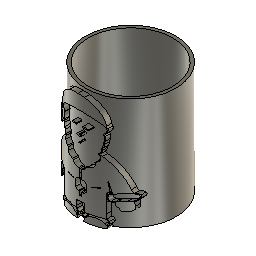
BICCHIERE BABBO NATALE v4 (Autodesk Fusion 360 design; units mm, degrees)
Autodesk Fusion 360 part; units mm, degrees
note: some values were not read from the file. Set by a fixed rule: which face or edge a step refers to.
(part 1 of 2)
sketch "Schizzo1" plane through (0, 0, 0) normal (0, 1, 0) x (1, 0, 0)
  spline S0 degree 3 poles (3.8329, -102.7667) (12.4583, -100.5971) (18.8877, -93.5063) (20.1048, -84.775) knots 0 0 0 0 1 1 1 1
  spline S1 degree 3 poles (20.1048, -84.775) (20.2635, -83.6902) (20.5281, -82.7377) (20.6869, -82.6319) knots 0 0 0 0 1 1 1 1
  spline S2 degree 3 poles (20.6869, -82.6319) (21.56, -82.1027) (21.0308, -79.7744) (19.7079, -78.2398) knots 0 0 0 0 1 1 1 1
  line L0 (19.7079, -78.2398) -> (18.7819, -77.155)
  line L1 (18.7819, -77.155) -> (19.1787, -75.885)
  spline S3 degree 3 poles (19.1787, -75.885) (19.6814, -74.2446) (19.6814, -73.4508) (19.2052, -72.0221) knots 0 0 0 0 1 1 1 1
  spline S4 degree 3 poles (19.2052, -72.0221) (18.9935, -71.3871) (18.7819, -70.17) (18.7554, -69.2969) knots 0 0 0 0 1 1 1 1
  spline S5 degree 3 poles (18.7554, -69.2969) (18.7289, -68.2121) (18.4908, -67.286) (18.041, -66.3865) knots 0 0 0 0 1 1 1 1
  spline S6 degree 3 poles (18.041, -66.3865) (17.6442, -65.6456) (17.406, -64.6931) (17.4325, -64.1904) knots 0 0 0 0 1 1 1 1
  spline S7 degree 3 poles (17.4325, -64.1904) (17.4854, -63.1321) (16.6387, -61.1213) (15.9244, -60.6715) knots 0 0 0 0 1 1 1 1
  spline S8 degree 3 poles (15.9244, -60.6715) (15.4217, -60.354) (15.5539, -60.2481) (17.3796, -59.1633) knots 0 0 0 0 1 1 1 1
  spline S9 degree 3 poles (17.3796, -59.1633) (24.3117, -55.1152) (29.9737, -45.9871) (33.1752, -33.7104) knots 0 0 0 0 1 1 1 1
  spline S10 degree 3 poles (33.1752, -33.7104) (33.8896, -31.0381) (34.1277, -30.4296) (34.4981, -30.4825) knots 0 0 0 0 1 1 1 1
  spline S11 degree 3 poles (34.4981, -30.4825) (35.1596, -30.6148) (36.3767, -29.6094) (36.9058, -28.551) knots 0 0 0 0 1 1 1 1
  spline S12 degree 3 poles (36.9058, -28.551) (37.4879, -27.2546) (37.2233, -25.72) (36.2179, -24.6881) knots 0 0 0 0 1 1 1 1
  spline S13 degree 3 poles (36.2179, -24.6881) (35.53, -23.9738) (35.1331, -23.7885) (34.551, -23.8944) knots 0 0 0 0 1 1 1 1
  spline S14 degree 3 poles (34.551, -23.8944) (34.4187, -23.9208) (34.3923, -23.4975) (34.4717, -22.9419) knots 0 0 0 0 1 1 1 1
  spline S15 degree 3 poles (34.4717, -22.9419) (34.5775, -22.3863) (34.7098, -20.9575) (34.8156, -19.7669) knots 0 0 0 0 1 1 1 1
  spline S16 degree 3 poles (34.8156, -19.7669) (35.0802, -16.5125) (34.6304, -16.0627) (30.6087, -15.5865) knots 0 0 0 0 1 1 1 1
  spline S17 degree 3 poles (30.6087, -15.5865) (29.18, -15.4277) (29.0477, -15.4542) (28.3333, -16.1685) knots 0 0 0 0 1 1 1 1
  spline S18 degree 3 poles (28.3333, -16.1685) (27.8571, -16.6448) (27.5131, -17.3592) (27.3808, -18.0471) knots 0 0 0 0 1 1 1 1
  spline S19 degree 3 poles (27.3808, -18.0471) (27.2485, -18.8938) (27.0898, -19.1583) (26.7194, -19.1583) knots 0 0 0 0 1 1 1 1
  spline S20 degree 3 poles (26.7194, -19.1583) (26.005, -19.1583) (25.3964, -20.1638) (25.3964, -21.4073) knots 0 0 0 0 1 1 1 1
  spline S21 degree 3 poles (25.3964, -21.4073) (25.3964, -22.5715) (25.0525, -23.3652) (24.7614, -22.889) knots 0 0 0 0 1 1 1 1
  spline S22 degree 3 poles (24.7614, -22.889) (24.5233, -22.4921) (23.0152, -22.5185) (22.195, -22.9154) knots 0 0 0 0 1 1 1 1
  spline S23 degree 3 poles (22.195, -22.9154) (20.6075, -23.6563) (19.8931, -26.1698) (20.7662, -27.8896) knots 0 0 0 0 1 1 1 1
  spline S24 degree 3 poles (20.7662, -27.8896) (21.2425, -28.8156) (22.3802, -29.7417) (23.0417, -29.7417) knots 0 0 0 0 1 1 1 1
  spline S25 degree 3 poles (23.0417, -29.7417) (23.3327, -29.7417) (23.5444, -29.8475) (23.5444, -30.0063) knots 0 0 0 0 1 1 1 1
  spline S26 degree 3 poles (23.5444, -30.0063) (23.5444, -30.4031) (22.5125, -34.7688) (21.9304, -36.7531) knots 0 0 0 0 1 1 1 1
  spline S27 degree 3 poles (21.9304, -36.7531) (21.0837, -39.7165) (21.0837, -39.69) (21.3748, -39.399) knots 0 0 0 0 1 1 1 1
  spline S28 degree 3 poles (21.3748, -39.399) (21.6658, -39.1079) (22.6977, -35.536) (23.4385, -32.3081) knots 0 0 0 0 1 1 1 1
  spline S29 degree 3 poles (23.4385, -32.3081) (23.8619, -30.456) (23.9677, -30.2444) (24.4704, -30.3767) knots 0 0 0 0 1 1 1 1
  spline S30 degree 3 poles (24.4704, -30.3767) (25.9256, -30.7735) (29.6033, -31.1175) (31.376, -31.0117) knots 0 0 0 0 1 1 1 1
  spline S31 degree 3 poles (31.376, -31.0117) (32.7519, -30.9323) (33.3339, -30.9852) (33.3339, -31.1969) knots 0 0 0 0 1 1 1 1
  spline S32 degree 3 poles (33.3339, -31.1969) (33.3339, -31.726) (31.9581, -36.9913) (31.6935, -37.494) knots 0 0 0 0 1 1 1 1
  spline S33 degree 3 poles (31.6935, -37.494) (31.5612, -37.7585) (31.4025, -38.2348) (31.3496, -38.5523) knots 0 0 0 0 1 1 1 1
  spline S34 degree 3 poles (31.3496, -38.5523) (30.8469, -41.304) (25.2906, -51.9931) (24.5762, -51.5433) knots 0 0 0 0 1 1 1 1
  spline S35 degree 3 poles (24.5762, -51.5433) (24.4439, -51.464) (24.4175, -51.5698) (24.4969, -51.7815) knots 0 0 0 0 1 1 1 1
  spline S36 degree 3 poles (24.4969, -51.7815) (24.5762, -51.9931) (24.3646, -52.39) (23.9942, -52.6546) knots 0 0 0 0 1 1 1 1
  spline S37 degree 3 poles (23.9942, -52.6546) (23.6502, -52.9456) (23.3592, -53.2367) (23.3327, -53.3425) knots 0 0 0 0 1 1 1 1
  spline S38 degree 3 poles (23.3327, -53.3425) (23.2798, -53.4483) (22.7242, -54.1363) (22.0362, -54.8771) knots 0 0 0 0 1 1 1 1
  spline S39 degree 3 poles (22.0362, -54.8771) (20.3958, -56.6763) (18.0939, -58.4225) (17.6971, -58.1579) knots 0 0 0 0 1 1 1 1
  spline S40 degree 3 poles (17.6971, -58.1579) (17.5119, -58.0521) (17.4589, -58.0785) (17.5648, -58.2638) knots 0 0 0 0 1 1 1 1
  spline S41 degree 3 poles (17.5648, -58.2638) (17.6442, -58.4225) (17.5383, -58.6606) (17.2737, -58.8194) knots 0 0 0 0 1 1 1 1
  spline S42 degree 3 poles (17.2737, -58.8194) (16.8504, -59.031) (16.7975, -58.8988) (16.7975, -57.2848) knots 0 0 0 0 1 1 1 1
  spline S43 degree 3 poles (16.7975, -57.2848) (16.7975, -55.6973) (16.7181, -55.4063) (15.9508, -54.4538) knots 0 0 0 0 1 1 1 1
  spline S44 degree 3 poles (15.9508, -54.4538) (15.501, -53.8717) (14.6808, -53.1573) (14.0987, -52.8663) knots 0 0 0 0 1 1 1 1
  spline S45 degree 3 poles (14.0987, -52.8663) (13.1727, -52.39) (13.0933, -52.2577) (13.0669, -51.1729) knots 0 0 0 0 1 1 1 1
  spline S46 degree 3 poles (13.0669, -51.1729) (13.0669, -50.5115) (12.8552, -49.5325) (12.5906, -48.9769) knots 0 0 0 0 1 1 1 1
  spline S47 degree 3 poles (12.5906, -48.9769) (12.0614, -47.9185) (10.3681, -46.331) (9.9977, -46.5692) knots 0 0 0 0 1 1 1 1
  spline S48 degree 3 poles (9.9977, -46.5692) (9.8919, -46.6485) (9.786, -46.5692) (9.786, -46.4104) knots 0 0 0 0 1 1 1 1
  spline S49 degree 3 poles (9.786, -46.4104) (9.786, -46.2252) (9.6008, -46.1458) (9.3892, -46.2252) knots 0 0 0 0 1 1 1 1
  spline S50 degree 3 poles (9.3892, -46.2252) (9.1775, -46.331) (8.9394, -46.2781) (8.86, -46.1194) knots 0 0 0 0 1 1 1 1
  spline S51 degree 3 poles (8.86, -46.1194) (8.7542, -45.9871) (8.5689, -45.9342) (8.4367, -46.0135) knots 0 0 0 0 1 1 1 1
  spline S52 degree 3 poles (8.4367, -46.0135) (8.3044, -46.1194) (8.1985, -46.0665) (8.1985, -45.9342) knots 0 0 0 0 1 1 1 1
  spline S53 degree 3 poles (8.1985, -45.9342) (8.1985, -45.8019) (7.8281, -45.7225) (7.3783, -45.749) knots 0 0 0 0 1 1 1 1
  spline S54 degree 3 poles (7.3783, -45.749) (6.6904, -45.8019) (6.4787, -45.6696) (6.1083, -45.0346) knots 0 0 0 0 1 1 1 1
  spline S55 degree 3 poles (6.1083, -45.0346) (5.4469, -43.791) (4.3621, -42.7327) (3.1185, -42.0713) knots 0 0 0 0 1 1 1 1
  line L2 (3.1185, -42.0713) -> (1.9808, -41.4627)
  line L3 (1.9808, -41.4627) -> (1.9279, -37.7321)
  line L4 (1.9279, -37.7321) -> (1.875, -33.975)
  line L5 (1.875, -33.975) -> (2.6687, -33.975)
  spline S56 degree 3 poles (2.6687, -33.975) (3.8858, -33.975) (4.9706, -33.2871) (5.5527, -32.1229) knots 0 0 0 0 1 1 1 1
  line L6 (5.5527, -32.1229) -> (6.0819, -31.0646)
  line L7 (6.0819, -31.0646) -> (7.7487, -31.1969)
  line L8 (7.7487, -31.1969) -> (9.3892, -31.3027)
  line L9 (9.3892, -31.3027) -> (7.7223, -31.0381)
  line L10 (7.7223, -31.0381) -> (6.0554, -30.7471)
  line L11 (6.0554, -30.7471) -> (6.1612, -29.239)
  spline S57 degree 3 poles (6.1612, -29.239) (6.2142, -28.3923) (6.3464, -27.5721) (6.4787, -27.3604) knots 0 0 0 0 1 1 1 1
  spline S58 degree 3 poles (6.4787, -27.3604) (6.611, -27.1223) (6.5846, -27.0694) (6.3994, -27.2017) knots 0 0 0 0 1 1 1 1
  spline S59 degree 3 poles (6.3994, -27.2017) (6.2142, -27.3075) (6.0819, -27.2546) (6.0819, -27.0958) knots 0 0 0 0 1 1 1 1
  spline S60 degree 3 poles (6.0819, -27.0958) (6.0819, -26.7783) (7.8281, -26.8577) (10.6856, -27.2546) knots 0 0 0 0 1 1 1 1
  spline S61 degree 3 poles (10.6856, -27.2546) (14.6014, -27.8102) (18.9671, -29.186) (20.4223, -30.3238) knots 0 0 0 0 1 1 1 1
  spline S62 degree 3 poles (20.4223, -30.3238) (21.56, -31.1969) (21.8775, -31.9642) (21.3748, -32.5727) knots 0 0 0 0 1 1 1 1
  spline S63 degree 3 poles (21.3748, -32.5727) (21.1102, -32.9167) (21.1102, -32.9696) (21.3748, -32.8108) knots 0 0 0 0 1 1 1 1
  spline S64 degree 3 poles (21.3748, -32.8108) (21.6394, -32.6521) (21.6923, -32.7844) (21.5864, -33.3665) knots 0 0 0 0 1 1 1 1
  spline S65 degree 3 poles (21.5864, -33.3665) (21.5335, -33.7633) (21.4542, -34.266) (21.4542, -34.4513) knots 0 0 0 0 1 1 1 1
  spline S66 degree 3 poles (21.4542, -34.4513) (21.4277, -34.8481) (20.6075, -34.6894) (19.655, -34.0808) knots 0 0 0 0 1 1 1 1
  spline S67 degree 3 poles (19.655, -34.0808) (19.311, -33.8692) (18.9671, -33.7104) (18.8877, -33.7369) knots 0 0 0 0 1 1 1 1
  spline S68 degree 3 poles (18.8877, -33.7369) (18.7819, -33.7369) (18.6231, -33.631) (18.5437, -33.4988) knots 0 0 0 0 1 1 1 1
  spline S69 degree 3 poles (18.5437, -33.4988) (18.4644, -33.3665) (17.9617, -33.1813) (17.4589, -33.0754) knots 0 0 0 0 1 1 1 1
  spline S70 degree 3 poles (17.4589, -33.0754) (16.6387, -32.9167) (16.6652, -32.9696) (17.8558, -33.5252) knots 0 0 0 0 1 1 1 1
  spline S71 degree 3 poles (17.8558, -33.5252) (20.7398, -34.8481) (21.1631, -35.1392) (21.0573, -35.536) knots 0 0 0 0 1 1 1 1
  spline S72 degree 3 poles (21.0573, -35.536) (20.8192, -36.4092) (20.6604, -39.6635) (20.8721, -39.0021) knots 0 0 0 0 1 1 1 1
  spline S73 degree 3 poles (20.8721, -39.0021) (21.0044, -38.6317) (21.1367, -37.7585) (21.1367, -37.0177) knots 0 0 0 0 1 1 1 1
  spline S74 degree 3 poles (21.1367, -37.0177) (21.1631, -36.3033) (21.3483, -35.4831) (21.56, -35.1921) knots 0 0 0 0 1 1 1 1
  spline S75 degree 3 poles (21.56, -35.1921) (21.7452, -34.9275) (22.0098, -34.0808) (22.0892, -33.3135) knots 0 0 0 0 1 1 1 1
  spline S76 degree 3 poles (22.0892, -33.3135) (22.3008, -31.726) (21.851, -30.5883) (20.8192, -30.0327) knots 0 0 0 0 1 1 1 1
  spline S77 degree 3 poles (20.8192, -30.0327) (20.4223, -29.821) (20.2106, -29.5035) (20.29, -29.239) knots 0 0 0 0 1 1 1 1
  spline S78 degree 3 poles (20.29, -29.239) (20.3429, -29.0008) (20.2371, -28.3658) (20.0519, -27.8367) knots 0 0 0 0 1 1 1 1
  spline S79 degree 3 poles (20.0519, -27.8367) (19.7873, -27.0694) (19.7608, -25.6935) (19.9196, -21.7513) knots 0 0 0 0 1 1 1 1
  spline S80 degree 3 poles (19.9196, -21.7513) (20.0519, -18.9467) (20.0783, -14.7133) (19.9989, -12.3321) knots 0 0 0 0 1 1 1 1
  spline S81 degree 3 poles (19.9989, -12.3321) (19.8931, -9.3158) (19.9196, -8.0723) (20.1312, -8.1781) knots 0 0 0 0 1 1 1 1
  spline S82 degree 3 poles (20.1312, -8.1781) (20.4752, -8.4163) (21.3748, -7.6225) (21.8775, -6.6171) knots 0 0 0 0 1 1 1 1
  spline S83 degree 3 poles (21.8775, -6.6171) (22.4331, -5.5588) (22.1156, -4.2623) (21.1367, -3.4156) knots 0 0 0 0 1 1 1 1
  spline S84 degree 3 poles (21.1367, -3.4156) (20.3958, -2.8071) (20.3429, -2.6748) (20.6075, -1.9075) knots 0 0 0 0 1 1 1 1
  spline S85 degree 3 poles (20.6075, -1.9075) (21.2954, 0.024) (21.9304, -0.1083) (11.9292, -0.1083) knots 0 0 0 0 1 1 1 1
  line L12 (11.9292, -0.1083) -> (2.9598, -0.1083)
  line L13 (2.9598, -0.1083) -> (3.2244, -1.2196)
  spline S86 degree 3 poles (3.2244, -1.2196) (4.6002, -7.3579) (14.5485, -9.21) (19.2052, -4.1829) knots 0 0 0 0 1 1 1 1
  line L14 (19.2052, -4.1829) -> (20.3164, -2.9923)
  line L15 (20.3164, -2.9923) -> (20.8456, -3.7596)
  spline S87 degree 3 poles (20.8456, -3.7596) (21.6923, -4.9238) (21.7717, -5.691) (21.1631, -6.67) knots 0 0 0 0 1 1 1 1
  spline S88 degree 3 poles (21.1631, -6.67) (20.1577, -8.284) (19.4433, -8.4427) (11.9027, -8.4427) knots 0 0 0 0 1 1 1 1
  spline S89 degree 3 poles (11.9027, -8.4427) (4.5208, -8.4427) (4.1504, -8.3898) (2.9069, -6.8023) knots 0 0 0 0 1 1 1 1
  spline S90 degree 3 poles (2.9069, -6.8023) (2.2189, -5.9292) (2.3512, -4.8179) (3.2244, -3.8919) knots 0 0 0 0 1 1 1 1
  spline S91 degree 3 poles (3.2244, -3.8919) (3.6742, -3.4156) (3.7006, -3.2833) (3.3831, -3.2833) knots 0 0 0 0 1 1 1 1
  spline S92 degree 3 poles (3.3831, -3.2833) (2.7481, -3.2833) (2.0867, -4.2358) (1.9279, -5.3735) knots 0 0 0 0 1 1 1 1
  spline S93 degree 3 poles (1.9279, -5.3735) (1.7956, -6.3525) (1.875, -6.5377) (2.7481, -7.4108) knots 0 0 0 0 1 1 1 1
  line L16 (2.7481, -7.4108) -> (3.7271, -8.3898)
  line L17 (3.7271, -8.3898) -> (3.6477, -11.9617)
  line L18 (3.6477, -11.9617) -> (3.5683, -15.5071)
  line L19 (3.5683, -15.5071) -> (1.8485, -15.3748)
  spline S94 degree 3 poles (1.8485, -15.3748) (0.896, -15.3219) (-0.6121, -15.3483) (-1.5381, -15.4277) knots 0 0 0 0 1 1 1 1
  line L20 (-1.5381, -15.4277) -> (-3.1786, -15.6129)
  line L21 (-3.1786, -15.6129) -> (-3.1786, -13.999)
  spline S95 degree 3 poles (-3.1786, -13.999) (-3.1786, -13.1258) (-3.2579, -11.4325) (-3.3638, -10.2419) knots 0 0 0 0 1 1 1 1
  spline S96 degree 3 poles (-3.3638, -10.2419) (-3.4961, -8.3633) (-3.4696, -8.0458) (-3.0992, -8.0458) knots 0 0 0 0 1 1 1 1
  spline S97 degree 3 poles (-3.0992, -8.0458) (-2.5436, -8.0458) (-1.5911, -6.4319) (-1.5911, -5.4794) knots 0 0 0 0 1 1 1 1
  spline S98 degree 3 poles (-1.5911, -5.4794) (-1.5911, -4.6063) (-2.4642, -3.2833) (-3.0727, -3.2833) knots 0 0 0 0 1 1 1 1
  spline S99 degree 3 poles (-3.0727, -3.2833) (-3.5225, -3.2833) (-3.5225, -3.151) (-3.0463, -1.8281) knots 0 0 0 0 1 1 1 1
  spline S100 degree 3 poles (-3.0463, -1.8281) (-2.8346, -1.246) (-2.6758, -0.611) (-2.6494, -0.4523) knots 0 0 0 0 1 1 1 1
  spline S101 degree 3 poles (-2.6494, -0.4523) (-2.6494, -0.1877) (-4.7661, -0.1083) (-11.6452, -0.0554) knots 0 0 0 0 1 1 1 1
  line L22 (-11.6452, -0.0554) -> (-20.6411, 0.024)
  line L23 (-20.6411, 0.024) -> (-20.6411, -0.6375)
  spline S102 degree 3 poles (-20.6411, -0.6375) (-20.6411, -1.0079) (-20.4029, -1.7752) (-20.1383, -2.3838) knots 0 0 0 0 1 1 1 1
  spline S103 degree 3 poles (-20.1383, -2.3838) (-18.6567, -5.6381) (-14.2911, -7.649) (-10.0577, -6.961) knots 0 0 0 0 1 1 1 1
  spline S104 degree 3 poles (-10.0577, -6.961) (-7.7558, -6.5906) (-6.3536, -5.9292) (-4.7925, -4.474) knots 0 0 0 0 1 1 1 1
  line L24 (-4.7925, -4.474) -> (-3.4961, -3.2569)
  line L25 (-3.4961, -3.2569) -> (-2.8081, -4.0771)
  spline S105 degree 3 poles (-2.8081, -4.0771) (-1.6175, -5.5058) (-2.0408, -6.9346) (-3.9723, -7.94) knots 0 0 0 0 1 1 1 1
  spline S106 degree 3 poles (-3.9723, -7.94) (-4.7925, -8.3898) (-5.5598, -8.4427) (-11.2483, -8.4427) knots 0 0 0 0 1 1 1 1
  spline S107 degree 3 poles (-11.2483, -8.4427) (-14.7408, -8.4427) (-18.0481, -8.3369) (-18.5773, -8.231) knots 0 0 0 0 1 1 1 1
  spline S108 degree 3 poles (-18.5773, -8.231) (-19.1065, -8.1252) (-19.9002, -7.6754) (-20.35, -7.2785) knots 0 0 0 0 1 1 1 1
  spline S109 degree 3 poles (-20.35, -7.2785) (-21.3554, -6.3525) (-21.4613, -5.0296) (-20.6146, -3.9713) knots 0 0 0 0 1 1 1 1
  spline S110 degree 3 poles (-20.6146, -3.9713) (-20.2971, -3.5744) (-20.1383, -3.1775) (-20.2442, -3.0717) knots 0 0 0 0 1 1 1 1
  spline S111 degree 3 poles (-20.2442, -3.0717) (-20.5352, -2.7806) (-21.964, -4.6592) (-21.964, -5.3735) knots 0 0 0 0 1 1 1 1
  spline S112 degree 3 poles (-21.964, -5.3735) (-21.964, -6.1673) (-20.7733, -7.9665) (-20.1383, -8.1781) knots 0 0 0 0 1 1 1 1
  spline S113 degree 3 poles (-20.1383, -8.1781) (-19.715, -8.3104) (-19.6621, -8.9719) (-19.6621, -15.7188) knots 0 0 0 0 1 1 1 1
  spline S114 degree 3 poles (-19.6621, -15.7188) (-19.6356, -19.7933) (-19.5563, -24.0002) (-19.4769, -25.0585) knots 0 0 0 0 1 1 1 1
  line L26 (-19.4769, -25.0585) -> (-19.3181, -26.9635)
  line L27 (-19.3181, -26.9635) -> (-19.715, -25.9052)
  spline S115 degree 3 poles (-19.715, -25.9052) (-19.9267, -25.3231) (-20.1119, -24.8204) (-20.1119, -24.7675) knots 0 0 0 0 1 1 1 1
  spline S116 degree 3 poles (-20.1119, -24.7675) (-20.1119, -24.45) (-22.6519, -23.6298) (-23.1811, -23.7621) knots 0 0 0 0 1 1 1 1
  spline S117 degree 3 poles (-23.1811, -23.7621) (-24.1336, -24.0002) (-23.9483, -24.45) (-22.89, -24.45) knots 0 0 0 0 1 1 1 1
  spline S118 degree 3 poles (-22.89, -24.45) (-20.7469, -24.45) (-19.2388, -26.2492) (-19.8208, -28.1542) knots 0 0 0 0 1 1 1 1
  spline S119 degree 3 poles (-19.8208, -28.1542) (-19.9796, -28.6833) (-20.3765, -29.3713) (-20.694, -29.6623) knots 0 0 0 0 1 1 1 1
  spline S120 degree 3 poles (-20.694, -29.6623) (-21.6465, -30.5354) (-24.9008, -31.3556) (-28.1817, -31.5144) knots 0 0 0 0 1 1 1 1
  spline S121 degree 3 poles (-28.1817, -31.5144) (-33.4733, -31.779) (-35.4577, -30.8794) (-35.4577, -28.2335) knots 0 0 0 0 1 1 1 1
  spline S122 degree 3 poles (-35.4577, -28.2335) (-35.4577, -27.2281) (-35.3254, -26.9106) (-34.5317, -26.1169) knots 0 0 0 0 1 1 1 1
  spline S123 degree 3 poles (-34.5317, -26.1169) (-33.4998, -25.085) (-33.4469, -24.9792) (-33.9761, -24.9792) knots 0 0 0 0 1 1 1 1
  spline S124 degree 3 poles (-33.9761, -24.9792) (-34.1877, -24.9792) (-34.7169, -25.4025) (-35.1667, -25.9052) knots 0 0 0 0 1 1 1 1
  spline S125 degree 3 poles (-35.1667, -25.9052) (-35.8811, -26.7254) (-35.9869, -27.0429) (-35.9869, -28.2865) knots 0 0 0 0 1 1 1 1
  spline S126 degree 3 poles (-35.9869, -28.2865) (-35.9869, -29.5829) (-35.8811, -29.874) (-35.1402, -30.6677) knots 0 0 0 0 1 1 1 1
  spline S127 degree 3 poles (-35.1402, -30.6677) (-34.664, -31.1704) (-33.9761, -31.6202) (-33.6056, -31.6731) knots 0 0 0 0 1 1 1 1
  spline S128 degree 3 poles (-33.6056, -31.6731) (-32.9971, -31.779) (-32.8913, -32.0171) (-32.2298, -34.5306) knots 0 0 0 0 1 1 1 1
  spline S129 degree 3 poles (-32.2298, -34.5306) (-30.4306, -41.3833) (-27.9171, -47.2835) (-24.8479, -51.9138) knots 0 0 0 0 1 1 1 1
  spline S130 degree 3 poles (-24.8479, -51.9138) (-23.0488, -54.6125) (-19.9002, -57.9727) (-17.9158, -59.3485) knots 0 0 0 0 1 1 1 1
  spline S131 degree 3 poles (-17.9158, -59.3485) (-16.6988, -60.1688) (-16.6723, -60.2481) (-17.1486, -60.5921) knots 0 0 0 0 1 1 1 1
  spline S132 degree 3 poles (-17.1486, -60.5921) (-17.4396, -60.7773) (-17.81, -61.3065) (-17.9952, -61.7563) knots 0 0 0 0 1 1 1 1
  spline S133 degree 3 poles (-17.9952, -61.7563) (-18.1804, -62.1796) (-18.4186, -62.55) (-18.5508, -62.55) knots 0 0 0 0 1 1 1 1
  spline S134 degree 3 poles (-18.5508, -62.55) (-18.6831, -62.55) (-18.7625, -62.9998) (-18.7625, -63.5554) knots 0 0 0 0 1 1 1 1
  spline S135 degree 3 poles (-18.7625, -63.5554) (-18.7361, -64.1904) (-18.9742, -64.9842) (-19.4504, -65.8044) knots 0 0 0 0 1 1 1 1
  spline S136 degree 3 poles (-19.4504, -65.8044) (-20.059, -66.8627) (-20.1648, -67.3125) (-20.059, -68.3708) knots 0 0 0 0 1 1 1 1
  line L28 (-20.059, -68.3708) -> (-19.9267, -69.6673)
  line L29 (-19.9267, -69.6673) -> (-20.9321, -68.6619)
  spline S137 degree 3 poles (-20.9321, -68.6619) (-21.4613, -68.0798) (-22.1492, -67.5506) (-22.4402, -67.4713) knots 0 0 0 0 1 1 1 1
  spline S138 degree 3 poles (-22.4402, -67.4713) (-22.7577, -67.3654) (-23.0488, -66.9685) (-23.1546, -66.5452) knots 0 0 0 0 1 1 1 1
  spline S139 degree 3 poles (-23.1546, -66.5452) (-23.3398, -65.6192) (-24.8479, -64.0846) (-26.1444, -63.4496) knots 0 0 0 0 1 1 1 1
  spline S140 degree 3 poles (-26.1444, -63.4496) (-27.679, -62.7088) (-29.7692, -62.7881) (-31.3038, -63.6877) knots 0 0 0 0 1 1 1 1
  spline S141 degree 3 poles (-31.3038, -63.6877) (-33.8702, -65.1958) (-34.9815, -67.8417) (-34.2406, -70.6727) knots 0 0 0 0 1 1 1 1
  spline S142 degree 3 poles (-34.2406, -70.6727) (-33.7908, -72.3925) (-33.0236, -73.345) (-31.2244, -74.3504) knots 0 0 0 0 1 1 1 1
  spline S143 degree 3 poles (-31.2244, -74.3504) (-30.219, -74.9325) (-29.7692, -75.0119) (-28.3669, -74.9325) knots 0 0 0 0 1 1 1 1
  spline S144 degree 3 poles (-28.3669, -74.9325) (-27.3615, -74.8796) (-26.5942, -74.6944) (-26.4619, -74.4827) knots 0 0 0 0 1 1 1 1
  spline S145 degree 3 poles (-26.4619, -74.4827) (-26.0915, -73.8742) (-25.2713, -76.6788) (-24.1336, -82.3938) knots 0 0 0 0 1 1 1 1
  spline S146 degree 3 poles (-24.1336, -82.3938) (-22.7577, -89.3258) (-22.255, -90.8869) (-20.6675, -93.2681) knots 0 0 0 0 1 1 1 1
  spline S147 degree 3 poles (-20.6675, -93.2681) (-18.4715, -96.6283) (-15.3758, -99.2477) (-11.3277, -101.1792) knots 0 0 0 0 1 1 1 1
  spline S148 degree 3 poles (-11.3277, -101.1792) (-8.0204, -102.7667) (-6.4858, -103.0842) (-2.1202, -103.19) knots 0 0 0 0 1 1 1 1
  spline S149 degree 3 poles (-2.1202, -103.19) (1.0548, -103.2694) (2.0867, -103.19) (3.8329, -102.7667) knots 0 0 0 0 1 1 1 1
  spline S150 degree 3 poles (-5.8773, -102.6079) (-8.4967, -102.1052) (-12.0156, -100.65) (-14.3969, -99.036) knots 0 0 0 0 1 1 1 1
  spline S151 degree 3 poles (-14.3969, -99.036) (-18.2333, -96.4696) (-21.6465, -92.0246) (-22.3608, -88.7438) knots 0 0 0 0 1 1 1 1
  spline S152 degree 3 poles (-22.3608, -88.7438) (-22.3873, -88.5321) (-22.5725, -87.8706) (-22.7048, -87.2885) knots 0 0 0 0 1 1 1 1
  spline S153 degree 3 poles (-22.7048, -87.2885) (-22.8636, -86.7065) (-23.0488, -85.9392) (-23.1281, -85.5688) knots 0 0 0 0 1 1 1 1
  spline S154 degree 3 poles (-23.1281, -85.5688) (-23.1811, -85.1983) (-23.3133, -84.6163) (-23.3927, -84.2458) knots 0 0 0 0 1 1 1 1
  spline S155 degree 3 poles (-23.3927, -84.2458) (-23.4721, -83.8754) (-23.5779, -83.2404) (-23.6573, -82.7906) knots 0 0 0 0 1 1 1 1
  spline S156 degree 3 poles (-23.6573, -82.7906) (-23.8954, -81.1502) (-24.8479, -77.0756) (-25.2713, -75.8056) knots 0 0 0 0 1 1 1 1
  line L30 (-25.2713, -75.8056) -> (-25.6946, -74.4827)
  line L31 (-25.6946, -74.4827) -> (-24.5833, -73.4773)
  spline S157 degree 3 poles (-24.5833, -73.4773) (-23.2604, -72.2867) (-22.5196, -70.7521) (-22.4931, -69.244) knots 0 0 0 0 1 1 1 1
  spline S158 degree 3 poles (-22.4931, -69.244) (-22.4931, -68.2915) (-22.4402, -68.1592) (-21.964, -68.2915) knots 0 0 0 0 1 1 1 1
  spline S159 degree 3 poles (-21.964, -68.2915) (-21.6729, -68.3708) (-21.1702, -68.7942) (-20.8792, -69.2175) knots 0 0 0 0 1 1 1 1
  spline S160 degree 3 poles (-20.8792, -69.2175) (-20.35, -69.9319) (-20.35, -70.0377) (-20.7469, -71.0431) knots 0 0 0 0 1 1 1 1
  spline S161 degree 3 poles (-20.7469, -71.0431) (-21.329, -72.4719) (-21.2761, -74.4298) (-20.6411, -76.0967) knots 0 0 0 0 1 1 1 1
  line L32 (-20.6411, -76.0967) -> (-20.1119, -77.4725)
  line L33 (-20.1119, -77.4725) -> (-20.9056, -78.2927)
  spline S162 degree 3 poles (-20.9056, -78.2927) (-21.7788, -79.1923) (-22.2021, -81.1238) (-21.8581, -82.5525) knots 0 0 0 0 1 1 1 1
  spline S163 degree 3 poles (-21.8581, -82.5525) (-21.6994, -83.161) (-18.789, -86.389) (-18.789, -85.9656) knots 0 0 0 0 1 1 1 1
  spline S164 degree 3 poles (-18.789, -85.9656) (-18.789, -85.9127) (-17.8629, -86.3096) (-16.7517, -86.8652) knots 0 0 0 0 1 1 1 1
  spline S165 degree 3 poles (-16.7517, -86.8652) (-11.4336, -89.511) (-6.8033, -90.6752) (-1.5911, -90.7017) knots 0 0 0 0 1 1 1 1
  spline S166 degree 3 poles (-1.5911, -90.7017) (5.1029, -90.7546) (10.3946, -89.5375) (15.8979, -86.7065) knots 0 0 0 0 1 1 1 1
  spline S167 degree 3 poles (15.8979, -86.7065) (17.2737, -86.0185) (18.5437, -85.4629) (18.7025, -85.4894) knots 0 0 0 0 1 1 1 1
  spline S168 degree 3 poles (18.7025, -85.4894) (18.8877, -85.4894) (18.9671, -85.41) (18.9142, -85.2777) knots 0 0 0 0 1 1 1 1
  spline S169 degree 3 poles (18.9142, -85.2777) (18.8348, -85.1719) (19.02, -84.9338) (19.311, -84.775) knots 0 0 0 0 1 1 1 1
  spline S170 degree 3 poles (19.311, -84.775) (19.9196, -84.4575) (19.9196, -84.3517) (19.2581, -87.024) knots 0 0 0 0 1 1 1 1
  spline S171 degree 3 poles (19.2581, -87.024) (18.676, -89.4581) (16.8504, -93.5063) (16.3212, -93.5063) knots 0 0 0 0 1 1 1 1
  spline S172 degree 3 poles (16.3212, -93.5063) (16.2154, -93.5063) (16.136, -93.665) (16.136, -93.8767) knots 0 0 0 0 1 1 1 1
  spline S173 degree 3 poles (16.136, -93.8767) (16.136, -94.2471) (12.5642, -98.0042) (11.3735, -98.8773) knots 0 0 0 0 1 1 1 1
  spline S174 degree 3 poles (11.3735, -98.8773) (11.0031, -99.1683) (10.2887, -99.5652) (9.786, -99.8033) knots 0 0 0 0 1 1 1 1
  spline S175 degree 3 poles (9.786, -99.8033) (9.2833, -100.0679) (8.8071, -100.3325) (8.7277, -100.4119) knots 0 0 0 0 1 1 1 1
  spline S176 degree 3 poles (8.7277, -100.4119) (8.1985, -100.994) (4.2298, -102.3698) (1.9014, -102.7667) knots 0 0 0 0 1 1 1 1
  spline S177 degree 3 poles (1.9014, -102.7667) (-0.0829, -103.0842) (-3.6813, -103.0313) (-5.8773, -102.6079) knots 0 0 0 0 1 1 1 1
  spline S178 degree 3 poles (-6.6975, -89.6698) (-10.9308, -88.929) (-17.6248, -86.2038) (-19.8738, -84.2988) knots 0 0 0 0 1 1 1 1
  spline S179 degree 3 poles (-19.8738, -84.2988) (-22.2286, -82.3408) (-21.8317, -78.9277) (-19.1065, -77.7371) knots 0 0 0 0 1 1 1 1
  spline S180 degree 3 poles (-19.1065, -77.7371) (-19.0536, -77.7106) (-19.3181, -77.2608) (-19.6886, -76.7317) knots 0 0 0 0 1 1 1 1
  spline S181 degree 3 poles (-19.6886, -76.7317) (-20.7733, -75.1177) (-20.9056, -72.6835) (-20.0325, -70.6992) knots 0 0 0 0 1 1 1 1
  spline S182 degree 3 poles (-20.0325, -70.6992) (-19.8208, -70.2229) (-19.5827, -69.1381) (-19.5033, -68.2915) knots 0 0 0 0 1 1 1 1
  spline S183 degree 3 poles (-19.5033, -68.2915) (-19.3975, -67.3654) (-19.08, -66.3071) (-18.6831, -65.5398) knots 0 0 0 0 1 1 1 1
  spline S184 degree 3 poles (-18.6831, -65.5398) (-18.3127, -64.8783) (-17.9952, -64.0581) (-17.9952, -63.7142) knots 0 0 0 0 1 1 1 1
  spline S185 degree 3 poles (-17.9952, -63.7142) (-17.9952, -62.7617) (-17.5719, -61.915) (-16.7252, -61.0948) knots 0 0 0 0 1 1 1 1
  line L34 (-16.7252, -61.0948) -> (-15.9315, -60.354)
  line L35 (-15.9315, -60.354) -> (-16.6988, -59.4015)
  spline S186 degree 3 poles (-16.6988, -59.4015) (-17.6777, -58.1844) (-17.8894, -57.0731) (-17.3867, -55.8825) knots 0 0 0 0 1 1 1 1
  spline S187 degree 3 poles (-17.3867, -55.8825) (-16.9369, -54.8242) (-15.5081, -53.5806) (-14.2381, -53.1308) knots 0 0 0 0 1 1 1 1
  spline S188 degree 3 poles (-14.2381, -53.1308) (-13.709, -52.9456) (-13.4179, -52.681) (-13.4708, -52.4694) knots 0 0 0 0 1 1 1 1
  spline S189 degree 3 poles (-13.4708, -52.4694) (-13.8148, -51.3846) (-13.7619, -50.1146) (-13.3915, -49.3738) knots 0 0 0 0 1 1 1 1
  spline S190 degree 3 poles (-13.3915, -49.3738) (-12.5713, -47.7863) (-9.9783, -46.4104) (-7.8088, -46.4104) knots 0 0 0 0 1 1 1 1
  spline S191 degree 3 poles (-7.8088, -46.4104) (-7.0679, -46.4104) (-6.9356, -46.3046) (-6.8033, -45.6431) knots 0 0 0 0 1 1 1 1
  spline S192 degree 3 poles (-6.8033, -45.6431) (-6.4594, -43.9763) (-4.3427, -42.4152) (-1.8556, -42.0448) knots 0 0 0 0 1 1 1 1
  line L36 (-1.8556, -42.0448) -> (-0.665, -41.886)
  line L37 (-0.665, -41.886) -> (-0.7444, -37.785)
  line L38 (-0.7444, -37.785) -> (-0.8238, -33.7104)
  line L39 (-0.8238, -33.7104) -> (-1.6969, -33.7104)
  spline S193 degree 3 poles (-1.6969, -33.7104) (-2.8346, -33.7104) (-4.2369, -32.7579) (-4.8454, -31.5938) knots 0 0 0 0 1 1 1 1
  spline S194 degree 3 poles (-4.8454, -31.5938) (-5.4804, -30.3502) (-5.3746, -26.2227) (-4.6867, -25.1379) knots 0 0 0 0 1 1 1 1
  spline S195 degree 3 poles (-4.6867, -25.1379) (-4.0517, -24.159) (-2.7023, -23.3917) (-1.6704, -23.3917) knots 0 0 0 0 1 1 1 1
  line L40 (-1.6704, -23.3917) -> (-0.7973, -23.3917)
  line L41 (-0.7973, -23.3917) -> (-0.7973, -21.7248)
  line L42 (-0.7973, -21.7248) -> (-0.7973, -20.0579)
  line L43 (-0.7973, -20.0579) -> (0.1287, -20.0315)
  line L44 (0.1287, -20.0315) -> (1.0548, -20.005)
  line L45 (1.0548, -20.005) -> (1.0548, -21.6983)
  line L46 (1.0548, -21.6983) -> (1.0548, -23.3917)
  line L47 (1.0548, -23.3917) -> (2.0073, -23.3917)
  spline S196 degree 3 poles (2.0073, -23.3917) (3.3037, -23.3917) (4.9177, -24.3442) (5.4204, -25.4025) knots 0 0 0 0 1 1 1 1
  spline S197 degree 3 poles (5.4204, -25.4025) (6.0025, -26.6725) (5.976, -30.6677) (5.341, -31.8319) knots 0 0 0 0 1 1 1 1
  spline S198 degree 3 poles (5.341, -31.8319) (4.7325, -32.9431) (3.3831, -33.7104) (2.0602, -33.7104) knots 0 0 0 0 1 1 1 1
  line L48 (2.0602, -33.7104) -> (1.0548, -33.7104)
  line L49 (1.0548, -33.7104) -> (1.0548, -37.8908)
  line L50 (1.0548, -37.8908) -> (1.0548, -42.0977)
  line L51 (1.0548, -42.0977) -> (2.1396, -42.4152)
  spline S199 degree 3 poles (2.1396, -42.4152) (3.4889, -42.8385) (5.1823, -44.3202) (5.5527, -45.5108) knots 0 0 0 0 1 1 1 1
  spline S200 degree 3 poles (5.5527, -45.5108) (5.7908, -46.2517) (6.0025, -46.4104) (6.5846, -46.4104) knots 0 0 0 0 1 1 1 1
  spline S201 degree 3 poles (6.5846, -46.4104) (8.1721, -46.4104) (10.1564, -47.2571) (11.2942, -48.3948) knots 0 0 0 0 1 1 1 1
  spline S202 degree 3 poles (11.2942, -48.3948) (12.326, -49.4267) (12.4319, -49.6383) (12.4319, -50.8554) knots 0 0 0 0 1 1 1 1
  spline S203 degree 3 poles (12.4319, -50.8554) (12.4319, -51.5963) (12.2996, -52.2842) (12.1408, -52.39) knots 0 0 0 0 1 1 1 1
  spline S204 degree 3 poles (12.1408, -52.39) (11.9821, -52.4694) (12.5642, -52.8927) (13.4637, -53.3425) knots 0 0 0 0 1 1 1 1
  spline S205 degree 3 poles (13.4637, -53.3425) (14.3369, -53.7658) (15.3158, -54.4538) (15.6333, -54.9035) knots 0 0 0 0 1 1 1 1
  spline S206 degree 3 poles (15.6333, -54.9035) (16.7446, -56.4646) (16.5329, -58.449) (15.1306, -59.7454) knots 0 0 0 0 1 1 1 1
  line L52 (15.1306, -59.7454) -> (14.575, -60.2217)
  line L53 (14.575, -60.2217) -> (15.3423, -60.8567)
  spline S207 degree 3 poles (15.3423, -60.8567) (16.3742, -61.7298) (17.0356, -63.529) (16.6917, -64.4815) knots 0 0 0 0 1 1 1 1
  spline S208 degree 3 poles (16.6917, -64.4815) (16.5064, -64.9313) (16.5064, -65.2223) (16.6917, -65.3281) knots 0 0 0 0 1 1 1 1
  spline S209 degree 3 poles (16.6917, -65.3281) (17.3531, -65.7515) (18.0675, -67.7888) (18.1204, -69.4292) knots 0 0 0 0 1 1 1 1
  spline S210 degree 3 poles (18.1204, -69.4292) (18.1204, -70.3817) (18.3056, -71.44) (18.4908, -71.784) knots 0 0 0 0 1 1 1 1
  spline S211 degree 3 poles (18.4908, -71.784) (18.9671, -72.6306) (18.9142, -75.1971) (18.4114, -76.4142) knots 0 0 0 0 1 1 1 1
  spline S212 degree 3 poles (18.4114, -76.4142) (17.9881, -77.4196) (17.9881, -77.4196) (18.8083, -78.081) knots 0 0 0 0 1 1 1 1
  spline S213 degree 3 poles (18.8083, -78.081) (20.8985, -79.8538) (20.8985, -82.5525) (18.7819, -84.3252) knots 0 0 0 0 1 1 1 1
  spline S214 degree 3 poles (18.7819, -84.3252) (16.6652, -86.1244) (9.8125, -88.8231) (5.3939, -89.6433) knots 0 0 0 0 1 1 1 1
  spline S215 degree 3 poles (5.3939, -89.6433) (2.5629, -90.146) (-3.8665, -90.1725) (-6.6975, -89.6698) knots 0 0 0 0 1 1 1 1
  spline S216 degree 3 poles (-29.9808, -74.1652) (-31.2244, -73.8213) (-32.8648, -72.3925) (-33.4733, -71.096) knots 0 0 0 0 1 1 1 1
  spline S217 degree 3 poles (-33.4733, -71.096) (-34.5846, -68.7677) (-33.394, -65.5133) (-30.9863, -64.2169) knots 0 0 0 0 1 1 1 1
  spline S218 degree 3 poles (-30.9863, -64.2169) (-26.2767, -61.7298) (-21.0644, -67.2331) (-23.8425, -71.731) knots 0 0 0 0 1 1 1 1
  spline S219 degree 3 poles (-23.8425, -71.731) (-25.1919, -73.9006) (-27.5467, -74.8531) (-29.9808, -74.1652) knots 0 0 0 0 1 1 1 1
  spline S220 degree 3 poles (-20.8792, -56.2265) (-22.1756, -54.8506) (-24.7686, -51.5169) (-25.5888, -50.1146) knots 0 0 0 0 1 1 1 1
  spline S221 degree 3 poles (-25.5888, -50.1146) (-27.9436, -46.1723) (-31.3831, -37.7056) (-31.145, -36.4356) knots 0 0 0 0 1 1 1 1
  spline S222 degree 3 poles (-31.145, -36.4356) (-31.0921, -36.1181) (-31.1186, -35.9065) (-31.2244, -35.9594) knots 0 0 0 0 1 1 1 1
  spline S223 degree 3 poles (-31.2244, -35.9594) (-31.4096, -36.0652) (-31.8065, -34.7952) (-32.1769, -32.9431) knots 0 0 0 0 1 1 1 1
  line L54 (-32.1769, -32.9431) -> (-32.3356, -32.0435)
  line L55 (-32.3356, -32.0435) -> (-30.9333, -32.1758)
  spline S224 degree 3 poles (-30.9333, -32.1758) (-29.5575, -32.3081) (-26.6206, -32.1229) (-24.0542, -31.726) knots 0 0 0 0 1 1 1 1
  line L56 (-24.0542, -31.726) -> (-22.8371, -31.5408)
  line L57 (-22.8371, -31.5408) -> (-21.964, -35.0598)
  spline S225 degree 3 poles (-21.964, -35.0598) (-21.4877, -36.9913) (-21.0908, -38.7375) (-21.0908, -38.9227) knots 0 0 0 0 1 1 1 1
  spline S226 degree 3 poles (-21.0908, -38.9227) (-21.0908, -39.1344) (-20.985, -39.1873) (-20.8792, -39.0815) knots 0 0 0 0 1 1 1 1
  spline S227 degree 3 poles (-20.8792, -39.0815) (-20.7469, -38.9492) (-21.0644, -37.2029) (-21.5671, -35.1656) knots 0 0 0 0 1 1 1 1
  spline S228 degree 3 poles (-21.5671, -35.1656) (-22.5461, -31.1969) (-22.6254, -30.6942) (-22.255, -30.9323) knots 0 0 0 0 1 1 1 1
  spline S229 degree 3 poles (-22.255, -30.9323) (-22.0963, -31.0117) (-21.5671, -30.6942) (-21.0379, -30.2444) knots 0 0 0 0 1 1 1 1
  spline S230 degree 3 poles (-21.0379, -30.2444) (-20.5088, -29.7946) (-20.0325, -29.4771) (-19.9531, -29.53) knots 0 0 0 0 1 1 1 1
  spline S231 degree 3 poles (-19.9531, -29.53) (-19.9002, -29.6094) (-20.1119, -29.8475) (-20.4823, -30.0856) knots 0 0 0 0 1 1 1 1
  spline S232 degree 3 poles (-20.4823, -30.0856) (-21.7258, -30.9058) (-21.8846, -32.7844) (-20.9321, -35.4302) knots 0 0 0 0 1 1 1 1
  spline S233 degree 3 poles (-20.9321, -35.4302) (-20.7998, -35.88) (-20.5352, -36.8854) (-20.4029, -37.6792) knots 0 0 0 0 1 1 1 1
  line L58 (-20.4029, -37.6792) -> (-20.1383, -39.1344)
  line L59 (-20.1383, -39.1344) -> (-20.2442, -37.494)
  spline S234 degree 3 poles (-20.2442, -37.494) (-20.3236, -36.5944) (-20.4029, -35.7213) (-20.4294, -35.536) knots 0 0 0 0 1 1 1 1
  spline S235 degree 3 poles (-20.4294, -35.536) (-20.5352, -35.1127) (-18.6302, -34.0279) (-16.1431, -33.1283) knots 0 0 0 0 1 1 1 1
  spline S236 degree 3 poles (-16.1431, -33.1283) (-15.0583, -32.7315) (-14.3704, -32.414) (-14.635, -32.414) knots 0 0 0 0 1 1 1 1
  spline S237 degree 3 poles (-14.635, -32.414) (-14.8996, -32.3875) (-15.5081, -32.5727) (-16.0108, -32.7579) knots 0 0 0 0 1 1 1 1
  spline S238 degree 3 poles (-16.0108, -32.7579) (-16.5136, -32.9696) (-16.9369, -33.1019) (-16.9369, -33.049) knots 0 0 0 0 1 1 1 1
  spline S239 degree 3 poles (-16.9369, -33.049) (-16.9369, -32.996) (-17.7306, -33.34) (-18.7096, -33.8692) knots 0 0 0 0 1 1 1 1
  spline S240 degree 3 poles (-18.7096, -33.8692) (-19.6886, -34.3719) (-20.5617, -34.6894) (-20.6675, -34.5835) knots 0 0 0 0 1 1 1 1
  spline S241 degree 3 poles (-20.6675, -34.5835) (-21.0908, -34.1073) (-21.1967, -31.8054) (-20.7998, -31.2233) knots 0 0 0 0 1 1 1 1
  spline S242 degree 3 poles (-20.7998, -31.2233) (-20.4823, -30.7206) (-17.5719, -28.9479) (-16.8046, -28.7892) knots 0 0 0 0 1 1 1 1
  spline S243 degree 3 poles (-16.8046, -28.7892) (-16.6723, -28.7363) (-15.3494, -28.4188) (-13.8942, -28.0748) knots 0 0 0 0 1 1 1 1
  spline S244 degree 3 poles (-13.8942, -28.0748) (-10.19, -27.1752) (-8.5496, -26.8842) (-7.2267, -26.9371) knots 0 0 0 0 1 1 1 1
  spline S245 degree 3 poles (-7.2267, -26.9371) (-6.5652, -26.9371) (-6.089, -26.8313) (-6.089, -26.6725) knots 0 0 0 0 1 1 1 1
  spline S246 degree 3 poles (-6.089, -26.6725) (-6.089, -25.8523) (-17.5454, -28.1806) (-18.6302, -29.239) knots 0 0 0 0 1 1 1 1
  spline S247 degree 3 poles (-18.6302, -29.239) (-18.9742, -29.5565) (-19.6621, -29.5565) (-19.4504, -29.2125) knots 0 0 0 0 1 1 1 1
  spline S248 degree 3 poles (-19.4504, -29.2125) (-19.3711, -29.0802) (-19.1858, -28.2865) (-19.0536, -27.4663) knots 0 0 0 0 1 1 1 1
  spline S249 degree 3 poles (-19.0536, -27.4663) (-18.8948, -26.5402) (-18.5773, -25.6935) (-18.2069, -25.2702) knots 0 0 0 0 1 1 1 1
  line L60 (-18.2069, -25.2702) -> (-17.5983, -24.6088)
  line L61 (-17.5983, -24.6088) -> (-18.2863, -25.0321)
  line L62 (-18.2863, -25.0321) -> (-18.9742, -25.4819)
  line L63 (-18.9742, -25.4819) -> (-19.1594, -22.9154)
  spline S250 degree 3 poles (-19.1594, -22.9154) (-19.3711, -19.8727) (-19.3446, -10.2948) (-19.1329, -9.4217) knots 0 0 0 0 1 1 1 1
  spline S251 degree 3 poles (-19.1329, -9.4217) (-19.0006, -8.8131) (-18.9213, -8.8131) (-17.3602, -8.9719) knots 0 0 0 0 1 1 1 1
  spline S252 degree 3 poles (-17.3602, -8.9719) (-14.9525, -9.2629) (-5.5333, -9.1835) (-4.7131, -8.866) knots 0 0 0 0 1 1 1 1
  spline S253 degree 3 poles (-4.7131, -8.866) (-3.7871, -8.5221) (-3.7077, -8.7602) (-3.7077, -12.4115) knots 0 0 0 0 1 1 1 1
  spline S254 degree 3 poles (-3.7077, -12.4115) (-3.7077, -14.5281) (-3.6019, -15.4806) (-3.3902, -15.6394) knots 0 0 0 0 1 1 1 1
  spline S255 degree 3 poles (-3.3902, -15.6394) (-2.8611, -15.9569) (3.4096, -15.9304) (3.7006, -15.5865) knots 0 0 0 0 1 1 1 1
  spline S256 degree 3 poles (3.7006, -15.5865) (3.8329, -15.4277) (3.9652, -14.0783) (3.9917, -12.5702) knots 0 0 0 0 1 1 1 1
  spline S257 degree 3 poles (3.9917, -12.5702) (4.0181, -11.0621) (4.1239, -9.501) (4.2298, -9.1306) knots 0 0 0 0 1 1 1 1
  spline S258 degree 3 poles (4.2298, -9.1306) (4.3621, -8.7602) (4.4679, -8.575) (4.4679, -8.7073) knots 0 0 0 0 1 1 1 1
  spline S259 degree 3 poles (4.4679, -8.7073) (4.4944, -8.866) (4.7589, -8.9983) (5.0764, -9.0248) knots 0 0 0 0 1 1 1 1
  spline S260 degree 3 poles (5.0764, -9.0248) (5.8967, -9.0777) (17.0356, -9.0777) (18.385, -9.0248) knots 0 0 0 0 1 1 1 1
  line L64 (18.385, -9.0248) -> (19.4433, -8.9719)
  line L65 (19.4433, -8.9719) -> (19.5227, -13.7344)
  spline S261 degree 3 poles (19.5227, -13.7344) (19.6021, -18.3381) (19.3375, -26.1169) (19.1258, -25.1908) knots 0 0 0 0 1 1 1 1
  spline S262 degree 3 poles (19.1258, -25.1908) (19.0464, -24.9263) (18.8877, -24.7146) (18.7554, -24.7146) knots 0 0 0 0 1 1 1 1
  spline S263 degree 3 poles (18.7554, -24.7146) (18.6231, -24.7146) (18.6496, -24.9792) (18.8348, -25.2967) knots 0 0 0 0 1 1 1 1
  spline S264 degree 3 poles (18.8348, -25.2967) (19.1523, -25.9052) (20.1312, -29.2654) (19.9989, -29.3977) knots 0 0 0 0 1 1 1 1
  spline S265 degree 3 poles (19.9989, -29.3977) (19.9725, -29.4242) (19.0464, -29.1067) (17.9617, -28.6833) knots 0 0 0 0 1 1 1 1
  spline S266 degree 3 poles (17.9617, -28.6833) (15.6069, -27.7838) (11.5323, -26.9106) (8.4367, -26.6725) knots 0 0 0 0 1 1 1 1
  line L66 (8.4367, -26.6725) -> (6.2142, -26.4873)
  line L67 (6.2142, -26.4873) -> (5.6056, -25.2438)
  spline S267 degree 3 poles (5.6056, -25.2438) (4.9706, -23.9208) (3.8329, -23.1271) (2.5894, -23.1271) knots 0 0 0 0 1 1 1 1
  spline S268 degree 3 poles (2.5894, -23.1271) (1.7692, -23.1271) (1.5046, -22.889) (1.875, -22.4392) knots 0 0 0 0 1 1 1 1
  spline S269 degree 3 poles (1.875, -22.4392) (2.0602, -22.2275) (2.0602, -22.0688) (1.8485, -21.9365) knots 0 0 0 0 1 1 1 1
  spline S270 degree 3 poles (1.8485, -21.9365) (1.7162, -21.8571) (1.5839, -21.6454) (1.5839, -21.5131) knots 0 0 0 0 1 1 1 1
  spline S271 degree 3 poles (1.5839, -21.5131) (1.5839, -21.3544) (1.6898, -21.3279) (1.8485, -21.4073) knots 0 0 0 0 1 1 1 1
  spline S272 degree 3 poles (1.8485, -21.4073) (1.9808, -21.4867) (2.1131, -21.4602) (2.1131, -21.3015) knots 0 0 0 0 1 1 1 1
  spline S273 degree 3 poles (2.1131, -21.3015) (2.1131, -21.1692) (1.9808, -20.9575) (1.8221, -20.8781) knots 0 0 0 0 1 1 1 1
  spline S274 degree 3 poles (1.8221, -20.8781) (1.6633, -20.7723) (1.6104, -20.5077) (1.6898, -20.296) knots 0 0 0 0 1 1 1 1
  spline S275 degree 3 poles (1.6898, -20.296) (1.875, -19.8463) (0.4462, -19.1583) (-0.2946, -19.3435) knots 0 0 0 0 1 1 1 1
  spline S276 degree 3 poles (-1.4058, -21.6719) (-1.4058, -22.9683) (-1.4588, -23.1271) (-1.935, -23.1271) knots 0 0 0 0 1 1 1 1
  spline S277 degree 3 poles (-1.935, -23.1271) (-3.4431, -23.1271) (-5.3746, -24.7146) (-5.3746, -25.9317) knots 0 0 0 0 1 1 1 1
  spline S278 degree 3 poles (-5.3746, -25.9317) (-5.3746, -26.1169) (-5.454, -26.3021) (-5.5333, -26.3021) knots 0 0 0 0 1 1 1 1
  spline S279 degree 3 poles (-5.5333, -26.3021) (-5.6127, -26.3021) (-5.6392, -27.334) (-5.5863, -28.5775) knots 0 0 0 0 1 1 1 1
  spline S280 degree 3 poles (-5.5863, -28.5775) (-5.5069, -30.6148) (-5.5598, -30.8529) (-5.9302, -30.7206) knots 0 0 0 0 1 1 1 1
  spline S281 degree 3 poles (-5.9302, -30.7206) (-6.1948, -30.6148) (-6.3536, -30.6942) (-6.3536, -30.9323) knots 0 0 0 0 1 1 1 1
  spline S282 degree 3 poles (-6.3536, -30.9323) (-6.3536, -31.144) (-6.1948, -31.2498) (-5.9831, -31.1704) knots 0 0 0 0 1 1 1 1
  spline S283 degree 3 poles (-5.9831, -31.1704) (-5.7715, -31.091) (-5.3746, -31.4615) (-4.9248, -32.2023) knots 0 0 0 0 1 1 1 1
  spline S284 degree 3 poles (-4.9248, -32.2023) (-4.2369, -33.3929) (-3.2579, -33.975) (-1.935, -33.975) knots 0 0 0 0 1 1 1 1
  line L68 (-1.935, -33.975) -> (-1.3, -33.975)
  line L69 (-1.3, -33.975) -> (-1.3794, -37.6263)
  spline S285 degree 3 poles (-1.3794, -37.6263) (-1.4588, -40.8013) (-1.5117, -41.251) (-1.9086, -41.251) knots 0 0 0 0 1 1 1 1
  spline S286 degree 3 poles (-1.9086, -41.251) (-2.1467, -41.251) (-2.4377, -41.3569) (-2.5436, -41.4627) knots 0 0 0 0 1 1 1 1
  spline S287 degree 3 poles (-2.5436, -41.4627) (-2.6494, -41.5685) (-3.0198, -41.6479) (-3.3902, -41.6479) knots 0 0 0 0 1 1 1 1
  spline S288 degree 3 poles (-3.3902, -41.6479) (-4.5279, -41.6479) (-6.1683, -43.0502) (-7.2267, -44.8758) knots 0 0 0 0 1 1 1 1
  spline S289 degree 3 poles (-7.2267, -44.8758) (-7.6765, -45.696) (-7.8881, -45.8813) (-8.4438, -45.8019) knots 0 0 0 0 1 1 1 1
  spline S290 degree 3 poles (-8.4438, -45.8019) (-10.8779, -45.4579) (-14.2911, -48.3948) (-14.2911, -50.829) knots 0 0 0 0 1 1 1 1
  spline S291 degree 3 poles (-14.2911, -50.829) (-14.2911, -51.8873) (-14.7144, -52.7604) (-15.2171, -52.7604) knots 0 0 0 0 1 1 1 1
  spline S292 degree 3 poles (-15.2171, -52.7604) (-15.3229, -52.7604) (-15.8521, -53.1308) (-16.4077, -53.5542) knots 0 0 0 0 1 1 1 1
  spline S293 degree 3 poles (-16.4077, -53.5542) (-17.5983, -54.4802) (-18.3656, -56.2529) (-18.2069, -57.6288) knots 0 0 0 0 1 1 1 1
  line L70 (-18.2069, -57.6288) -> (-18.1011, -58.5283)
  line L71 (-18.1011, -58.5283) -> (-18.9213, -57.9992)
  spline S294 degree 3 poles (-18.9213, -57.9992) (-19.3446, -57.7081) (-20.2442, -56.9144) (-20.8792, -56.2265) knots 0 0 0 0 1 1 1 1
  spline S295 degree 3 poles (25.3964, -29.821) (24.3117, -29.6094) (23.0946, -29.2654) (22.6977, -29.0538) knots 0 0 0 0 1 1 1 1
  spline S296 degree 3 poles (22.6977, -29.0538) (20.2635, -27.8102) (20.2635, -24.4235) (22.7506, -23.3917) knots 0 0 0 0 1 1 1 1
  spline S297 degree 3 poles (22.7506, -23.3917) (23.5708, -23.0477) (23.9942, -23.1006) (26.5871, -23.7621) knots 0 0 0 0 1 1 1 1
  spline S298 degree 3 poles (26.5871, -23.7621) (27.6983, -24.0796) (29.1006, -24.1854) (31.376, -24.1325) knots 0 0 0 0 1 1 1 1
  spline S299 degree 3 poles (31.376, -24.1325) (35.0008, -24.0531) (35.7417, -24.3177) (36.4031, -25.9052) knots 0 0 0 0 1 1 1 1
  spline S300 degree 3 poles (36.4031, -25.9052) (37.1704, -27.7838) (35.9004, -29.8475) (33.7837, -30.1121) knots 0 0 0 0 1 1 1 1
  spline S301 degree 3 poles (33.7837, -30.1121) (33.1752, -30.1915) (32.3021, -30.3238) (31.8787, -30.3767) knots 0 0 0 0 1 1 1 1
  spline S302 degree 3 poles (31.8787, -30.3767) (30.6087, -30.5354) (27.5396, -30.2708) (25.3964, -29.821) knots 0 0 0 0 1 1 1 1
  spline S303 degree 3 poles (26.3754, -22.9948) (25.661, -22.8096) (25.6346, -22.7302) (25.7933, -21.6983) knots 0 0 0 0 1 1 1 1
  spline S304 degree 3 poles (25.7933, -21.6983) (26.0579, -19.9785) (26.1902, -19.714) (26.7723, -19.6346) knots 0 0 0 0 1 1 1 1
  spline S305 degree 3 poles (26.7723, -19.6346) (27.4337, -19.5288) (27.6719, -19.1583) (28.0423, -17.6502) knots 0 0 0 0 1 1 1 1
  spline S306 degree 3 poles (28.0423, -17.6502) (28.3862, -16.2479) (29.1271, -15.9569) (31.6935, -16.2479) knots 0 0 0 0 1 1 1 1
  spline S307 degree 3 poles (31.6935, -16.2479) (34.551, -16.5654) (34.6833, -16.8035) (34.26, -21.0633) knots 0 0 0 0 1 1 1 1
  spline S308 degree 3 poles (34.26, -21.0633) (34.0483, -23.1006) (34.0483, -23.1271) (33.2281, -23.2594) knots 0 0 0 0 1 1 1 1
  spline S309 degree 3 poles (33.2281, -23.2594) (31.2173, -23.5769) (28.2804, -23.471) (26.3754, -22.9948) knots 0 0 0 0 1 1 1 1
  spline S310 degree 3 poles (8.0927, -5.6646) (6.2671, -4.9767) (4.0975, -2.9129) (3.8329, -1.6429) knots 0 0 0 0 1 1 1 1
  spline S311 degree 3 poles (3.8329, -1.6429) (3.7271, -1.2196) (3.7006, -0.8227) (3.78, -0.7433) knots 0 0 0 0 1 1 1 1
  spline S312 degree 3 poles (3.78, -0.7433) (3.8329, -0.6904) (7.59, -0.5846) (12.1408, -0.5581) knots 0 0 0 0 1 1 1 1
  line L72 (12.1408, -0.5581) -> (20.3694, -0.5052)
  line L73 (20.3694, -0.5052) -> (20.3694, -1.1931)
  spline S313 degree 3 poles (20.3694, -1.1931) (20.3694, -2.0133) (18.6231, -4.1035) (17.1414, -5.0296) knots 0 0 0 0 1 1 1 1
  spline S314 degree 3 poles (17.1414, -5.0296) (14.7602, -6.5377) (11.0031, -6.8023) (8.0927, -5.6646) knots 0 0 0 0 1 1 1 1
  spline S315 degree 3 poles (-14.4233, -6.1408) (-15.905, -5.6646) (-17.3338, -4.7915) (-18.5773, -3.5479) knots 0 0 0 0 1 1 1 1
  spline S316 degree 3 poles (-18.5773, -3.5479) (-19.6356, -2.4896) (-20.4029, -1.0873) (-20.0854, -0.7698) knots 0 0 0 0 1 1 1 1
  spline S317 degree 3 poles (-20.0854, -0.7698) (-19.8738, -0.5846) (-19.0536, -0.5846) (-11.3277, -0.611) knots 0 0 0 0 1 1 1 1
  spline S318 degree 3 poles (-11.3277, -0.611) (-3.6019, -0.6375) (-3.4431, -0.6375) (-3.4431, -1.1667) knots 0 0 0 0 1 1 1 1
  spline S319 degree 3 poles (-3.4431, -1.1667) (-3.4431, -2.9658) (-6.7769, -5.691) (-9.6608, -6.2731) knots 0 0 0 0 1 1 1 1
  spline S320 degree 3 poles (-9.6608, -6.2731) (-10.6398, -6.4583) (-13.6296, -6.379) (-14.4233, -6.1408) knots 0 0 0 0 1 1 1 1
  spline S321 degree 3 poles (8.0927, -79.4833) (9.8389, -79.2188) (12.1673, -78.6896) (13.2521, -78.2927) knots 0 0 0 0 1 1 1 1
  spline S322 degree 3 poles (13.2521, -78.2927) (14.3369, -77.8958) (15.7656, -77.5254) (16.4535, -77.446) knots 0 0 0 0 1 1 1 1
  spline S323 degree 3 poles (16.4535, -77.446) (17.1679, -77.3667) (17.7235, -77.2079) (17.7235, -77.0756) knots 0 0 0 0 1 1 1 1
  spline S324 degree 3 poles (17.7235, -77.0756) (17.7235, -76.6258) (15.6069, -76.8375) (14.5485, -77.3667) knots 0 0 0 0 1 1 1 1
  spline S325 degree 3 poles (14.5485, -77.3667) (13.9664, -77.6577) (13.4637, -77.8958) (13.3844, -77.8958) knots 0 0 0 0 1 1 1 1
  spline S326 degree 3 poles (13.3844, -77.8958) (12.8287, -77.8958) (12.4848, -74.1123) (12.961, -73.001) knots 0 0 0 0 1 1 1 1
  spline S327 degree 3 poles (12.961, -73.001) (13.0933, -72.6571) (13.0139, -72.2073) (12.6964, -71.6781) knots 0 0 0 0 1 1 1 1
  spline S328 degree 3 poles (12.6964, -71.6781) (12.1144, -70.6992) (11.7969, -69.5085) (11.8762, -68.6619) knots 0 0 0 0 1 1 1 1
  spline S329 degree 3 poles (11.8762, -68.6619) (11.9556, -67.974) (11.9821, -67.9475) (9.1246, -68.7413) knots 0 0 0 0 1 1 1 1
  spline S330 degree 3 poles (9.1246, -68.7413) (8.2779, -68.9794) (6.5317, -69.1646) (5.2881, -69.191) knots 0 0 0 0 1 1 1 1
  spline S331 degree 3 poles (5.2881, -69.191) (3.436, -69.191) (3.145, -69.244) (3.7006, -69.4821) knots 0 0 0 0 1 1 1 1
  spline S332 degree 3 poles (3.7006, -69.4821) (4.706, -69.9054) (7.8546, -69.5879) (10.7385, -68.7413) knots 0 0 0 0 1 1 1 1
  spline S333 degree 3 poles (10.7385, -68.7413) (11.1883, -68.6354) (11.3471, -68.7413) (11.5058, -69.3498) knots 0 0 0 0 1 1 1 1
  spline S334 degree 3 poles (11.5058, -69.3498) (11.6381, -69.7467) (11.7439, -70.2758) (11.7439, -70.4875) knots 0 0 0 0 1 1 1 1
  spline S335 degree 3 poles (11.7439, -70.4875) (11.7704, -70.7256) (11.9556, -71.2019) (12.2202, -71.5723) knots 0 0 0 0 1 1 1 1
  spline S336 degree 3 poles (12.2202, -71.5723) (12.5642, -72.1279) (12.6171, -72.5513) (12.4319, -73.9535) knots 0 0 0 0 1 1 1 1
  spline S337 degree 3 poles (12.4319, -73.9535) (12.2996, -75.1442) (12.326, -75.9644) (12.5906, -76.7052) knots 0 0 0 0 1 1 1 1
  spline S338 degree 3 poles (12.5906, -76.7052) (12.9875, -77.9223) (12.9346, -78.0017) (10.9767, -78.425) knots 0 0 0 0 1 1 1 1
  spline S339 degree 3 poles (10.9767, -78.425) (7.2196, -79.2452) (3.4889, -79.5363) (-1.4588, -79.404) knots 0 0 0 0 1 1 1 1
  spline S340 degree 3 poles (-1.4588, -79.404) (-6.8298, -79.2452) (-9.4227, -78.9013) (-14.1852, -77.6313) knots 0 0 0 0 1 1 1 1
  spline S341 degree 3 poles (-14.1852, -77.6313) (-17.2808, -76.7846) (-18.3921, -76.6788) (-18.6567, -77.1021) knots 0 0 0 0 1 1 1 1
  spline S342 degree 3 poles (-18.6567, -77.1021) (-18.7625, -77.2608) (-18.4979, -77.3667) (-18.0481, -77.3667) knots 0 0 0 0 1 1 1 1
  spline S343 degree 3 poles (-18.0481, -77.3667) (-17.6248, -77.3667) (-15.6669, -77.7635) (-13.7354, -78.2663) knots 0 0 0 0 1 1 1 1
  spline S344 degree 3 poles (-13.7354, -78.2663) (-11.7775, -78.769) (-8.8406, -79.3775) (-7.2002, -79.5892) knots 0 0 0 0 1 1 1 1
  spline S345 degree 3 poles (-7.2002, -79.5892) (-3.1256, -80.1713) (3.9387, -80.1183) (8.0927, -79.4833) knots 0 0 0 0 1 1 1 1
  spline S346 degree 3 poles (6.2142, -78.3456) (7.0079, -78.081) (7.9339, -77.4196) (7.9339, -77.1285) knots 0 0 0 0 1 1 1 1
  spline S347 degree 3 poles (7.9339, -77.1285) (7.9339, -77.0492) (7.7487, -76.7581) (7.5371, -76.4671) knots 0 0 0 0 1 1 1 1
  spline S348 degree 3 poles (7.5371, -76.4671) (7.1931, -76.0173) (7.0873, -76.0173) (5.5527, -76.3877) knots 0 0 0 0 1 1 1 1
  spline S349 degree 3 poles (5.5527, -76.3877) (4.4414, -76.6788) (3.7271, -76.7317) (3.3037, -76.5729) knots 0 0 0 0 1 1 1 1